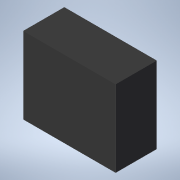
# Autodesk Inventor part: 13_Motor_Fixation_Thread_Mount
Saved by Autodesk Inventor 2021 (Build 250183000, 183)
## iProperties
Created: 2021-08-05
Part Number: 13_Motor_Fixation_Thread_Mount
Material: Generisch
Document SubType Name: Modeling
Designer: User
Density: 1 g/cm^3
Appearance: Vorgabe
Author: User
Autodesk Inventor part; units mm, degrees
ref_plane "YZ Plane" through (0, 0, 0) normal (1, 0, 0) x (0, 1, 0)
ref_plane "XZ Plane" through (0, 0, 0) normal (0, 1, 0) x (-1, 0, 0)
ref_plane "XY Plane" through (0, 0, 0) normal (0, 0, 1) x (1, 0, 0)
sketch "Skizze1" plane through (0, 0, 0) normal (0, 0, 1) x (1, 0, 0)
  line L0 (-41.9152, 0) -> (-41.9152, -12) projected
  line L1 (-53.9134, -12) -> (-41.9152, -12) projected
  line L2 (-53.9134, 0) -> (-53.9134, -12) projected
  line L3 (-41.9152, 0) -> (-53.9134, 0) projected
  line L4 (-39.4739, 0) -> (-39.4739, -12) projected
  line L5 (-41.9558, -12.0406) -> (-53.9549, -0.0415) construction
  line L6 (-53.9549, -11.9585) -> (-41.9558, 0.0406) construction
  circle A0 centre (-47.9553, -5.959) radius 1.675
  line L7 (-39.4739, -12) -> (-53.9134, -12)
  line L8 (-53.9134, -12) -> (-53.9134, 0)
  line L9 (-53.9134, 0) -> (-39.4739, 0)
  line L10 (-39.4739, 0) -> (-39.4739, -12)
  point P0 (0, 0)
  point P1 (-39.4739, 0)
  dimension "d0" = 3.35
  constraints: 10 end point, 2 parallel, 1 centre point, 1 horizontal, 1 perpendicular, 5 other
  measures "d0" diameter of A0
extrude "Extrusion1" add sketch "Skizze1" along normal blind 6.4 contours L9 L4 L7 L0 | L0 L1 L2 L3 | A0
sketch "Skizze2" plane through (0, 0, 0) normal (0, 0, -1) x (-1, 0, 0)
  circle A0 centre (47.9553, -5.959) radius 1.675 projected
  point P0 (0, 0)
extrude "Extrusion2" cut sketch "Skizze2" against normal blind 5.4
chamfer "Fase1" distance 0.6 angle 45 1 edges at (-46.2803, -5.959, 0)
